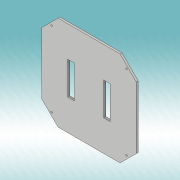
# Autodesk Inventor part: Middle_base
Saved by Autodesk Inventor 2019 (Build 230136000, 136)
## iProperties
Created: 2019-02-28
Part Number: Middle_base
Material: Generic
Document SubType Name: Modeling
Designer: USUARIO
Density: 1 g/cm^3
Appearance: Default
Author: USUARIO
Autodesk Inventor part; units mm, degrees
ref_plane "YZ Plane" through (0, 0, 0) normal (1, 0, 0) x (0, 1, 0)
ref_plane "XZ Plane" through (0, 0, 0) normal (0, 1, 0) x (-1, 0, 0)
ref_plane "XY Plane" through (0, 0, 0) normal (0, 0, 1) x (1, 0, 0)
sketch "Sketch1" plane through (0, 0, 0) normal (0, 0, 1) x (1, 0, 0)
  line L0 (0, 0) -> (-47.5, 0)
  line L1 (-47.5, 0) -> (-72.2487, 24.7487)
  line L2 (-72.2487, 24.7487) -> (-72.2487, 72.2487)
  line L3 (-72.2487, 72.2487) -> (0, 72.2487)
  line L4 (0, 72.2487) -> (0, 0)
  line L5 (0, 144.4975) -> (-47.5, 144.4975)
  line L6 (-47.5, 144.4975) -> (-72.2487, 119.7487)
  line L7 (-72.2487, 119.7487) -> (-72.2487, 72.2487)
  line L8 (0, 0) -> (47.5, 0)
  line L9 (47.5, 0) -> (72.2487, 24.7487)
  line L10 (72.2487, 24.7487) -> (72.2487, 72.2487)
  line L11 (72.2487, 119.7487) -> (72.2487, 72.2487)
  line L12 (47.5, 144.4975) -> (72.2487, 119.7487)
  line L13 (0, 144.4975) -> (47.5, 144.4975)
  dimension "d0" = 47.5
  dimension "d2" = 35
  dimension "d3" = 135
  constraints: 28 end point, 8 symmetric about line, 3 perpendicular, 2 horizontal
  measures "d0" distance of L0.start L0.end
  measures "d2" distance of L0.end L1.end
  measures "d3" angle of L0 L1
extrude "Extrusion1" add sketch "Sketch1" along normal mid plane 3
sketch "Sketch2" plane through (0, 0, 1.5) normal (0, 0, 1) x (1, 0, 0)
  line L0 (-32.5, 97.5) -> (-22.5, 97.5)
  line L1 (-22.5, 97.5) -> (-22.5, 47.5)
  line L2 (-22.5, 47.5) -> (-32.5, 47.5)
  line L3 (-32.5, 47.5) -> (-32.5, 97.5)
  line L4 (0, 0) -> (0, 144.4975)
  line L5 (-47.5, 144.4975) -> (47.5, 144.4975) projected
  line L6 (-47.5, 0) -> (47.5, 0) projected
  line L7 (32.5, 97.5) -> (22.5, 97.5)
  line L8 (22.5, 97.5) -> (22.5, 47.5)
  line L9 (22.5, 47.5) -> (32.5, 47.5)
  line L10 (32.5, 47.5) -> (32.5, 97.5)
  dimension "d6" = 50
  dimension "d7" = 10
  dimension "d8" = 45
  dimension "d10" = 47.5
  constraints: 18 end point, 4 symmetric about line, 2 parallel, 1 horizontal, 1 midpoint, 1 perpendicular
  measures "d6" distance of L2.end L0.start
  measures "d7" distance of L1.end L2.end
  measures "d8" diameter of L1 L4
  measures "d10" distance between parallel lines of L6 L2
extrude "Extrusion2" cut sketch "Sketch2" against normal blind 3
sketch "Sketch3" plane through (0, 0, 1.5) normal (0, 0, 1) x (1, 0, 0)
  line L0 (47.5, 144.4975) -> (-47.5, 144.4975) projected
  line L1 (0, 144.4975) -> (0, 0)
  line L2 (-72.2487, 119.7487) -> (-72.2487, 24.7487) projected
  line L3 (-72.2487, 72.2487) -> (0, 72.2487)
  circle A0 centre (-57.3995, 14.8492) radius 1.25
  line L4 (-72.2487, 24.7487) -> (-47.5, 0) projected
  line L5 (-59.8744, 12.3744) -> (0, 72.2487)
  circle A1 centre (-57.3995, 129.6482) radius 1.25
  circle A2 centre (57.3995, 14.8492) radius 1.25
  circle A3 centre (57.3995, 129.6482) radius 1.25
  dimension "d13" = 2.5
  dimension "d14" = 3.5
  constraints: 6 end point, 4 centre point, 4 midpoint, 3 symmetric about line, 1 point on line, 1 vertical, 3 other
  measures "d13" diameter of A0
  measures "d14" distance from line of A0.centre L4
extrude "Extrusion3" add sketch "Sketch3" along normal blind 0.1 contours L5 A0 | A0 L5 | A1 | A2 | A3
body "Solid1"
